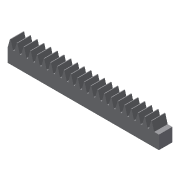
# Autodesk Inventor part: 00_gear_rack
Saved by Autodesk Inventor 2019.4 (Build 234330000, 330)
## iProperties
Created: 2021-02-14
Part Number: 00_gear_rack
Material: Generic
Document SubType Name: Modeling
Designer: diederichbenedict
Density: 1 g/cm^3
Appearance: Default
Author: diederichbenedict
Autodesk Inventor part; units mm, degrees
ref_plane "YZ Plane" through (0, 0, 0) normal (1, 0, 0) x (0, 1, 0)
ref_plane "XZ Plane" through (0, 0, 0) normal (0, 1, 0) x (-1, 0, 0)
ref_plane "XY Plane" through (0, 0, 0) normal (0, 0, 1) x (1, 0, 0)
sketch "Sketch1" plane through (0, 0, 0) normal (0, 0, 1) x (1, 0, 0)
  line L0 (0, 0) -> (-45, 0)
  line L1 (-45, 0) -> (-45, 4)
  line L2 (-45, 4) -> (0, 4)
  line L3 (0, 4) -> (0, 0)
  dimension "d0" = 45
  dimension "d1" = 4
  constraints: 8 end point, 2 parallel, 1 horizontal, 1 perpendicular
  measures "d0" distance of L1.end L2.end
  measures "d1" distance of L0.end L1.end
extrude "Extrusion1" add sketch "Sketch1" along normal blind 4
sketch "Sketch2" plane through (0, 0, 4) normal (0, 0, 1) x (1, 0, 0)
  line L0 (0, 4) -> (-45, 4) projected
  line L1 (-44.3, 6) -> (-44.2, 6)
  line L2 (-44.2, 6) -> (-44.2, 4)
  line L3 (-45, 4) -> (-44.2, 4)
  line L4 (-45, 4) -> (-44.3, 6)
  line L5 (-45, 4) -> (-45, 0) projected
  point P0 (0, 0)
  dimension "d4" = 0.1
  dimension "d10" = 0.8
  dimension "d11" = 2
  constraints: 8 end point, 1 collinear, 1 horizontal, 1 perpendicular, 1 point on line
  measures "d4" distance of L1.start L1.end
  measures "d10" distance between parallel lines of L2 L5
  measures "d11" distance between parallel lines of L0 L1
extrude "Extrusion2" add sketch "Sketch2" against normal up to surface (4 mm away)
mirror "Mirror1" about plane through (-44.2, 6, 4) normal (1, 0, 0) of "Extrusion2"
fillet "Fillet1" radius 0.2 3 edges at (-43.4, 4, 2) (-44.1, 6, 2) (-44.3, 6, 2)
pattern_linear "Rectangular Pattern2" count 22 spacing 2 along (1, 0, 0) of "Extrusion2", "Mirror1", "Fillet1"
body "Solid1"
